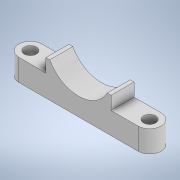
# Autodesk Inventor part: Стойка для заднего подшипника
Saved by Autodesk Inventor 2020 (Build 240168000, 168)
## iProperties
Created: 2021-04-13
Part Number: Стойка для заднего подшипника
Material: Типовые
Document SubType Name: Modeling
Designer: Антон
Density: 1 g/cm^3
Appearance: По умолчанию
Mass: 0.686339 g
Surface Area: 8.15331 cm^2
Volume: 0.686339 cm^3
Author: Антон
Autodesk Inventor part; units mm, degrees
ref_plane "YZ Plane" through (0, 0, 0) normal (1, 0, 0) x (0, 1, 0)
ref_plane "XZ Plane" through (0, 0, 0) normal (0, 1, 0) x (-1, 0, 0)
ref_plane "XY Plane" through (0, 0, 0) normal (0, 0, 1) x (1, 0, 0)
sketch "Эскиз6" plane through (0, 0, 0) normal (0, 0, 1) x (1, 0, 0)
  line L0 (0, 0) -> (10.05, 0)
  line L1 (10.05, 0) -> (10.05, 2)
  line L2 (10.05, 2) -> (0, 2)
  line L3 (0, 2) -> (0, 0)
  line L4 (10.05, 0) -> (27.05, 0)
  line L5 (27.05, 0) -> (27.05, 9.55)
  line L6 (27.05, 9.55) -> (10.05, 9.55)
  line L7 (10.05, 9.55) -> (10.05, 0)
  line L8 (27.05, 0) -> (37.1, 0)
  line L9 (37.1, 0) -> (37.1, 2)
  line L10 (37.1, 2) -> (27.05, 2)
  line L11 (27.05, 2) -> (27.05, 0)
  line L12 (10.05, 5.4448) -> (11.05, 5.4448)
  line L13 (27.05, 5.4448) -> (26.05, 5.4448)
  circle A0 centre (18.55, 9.55) radius 8.55
  line L14 (0, 0) -> (37.1, 0)
  line L15 (37.1, 0) -> (37.1, -3.7)
  line L16 (37.1, -3.7) -> (0, -3.7)
  line L17 (0, -3.7) -> (0, 0)
  point P0 (10.05, 2)
  dimension "d20" = 10.05
  dimension "d21" = 2
  dimension "d22" = 17
  dimension "d23" = 9.55
  dimension "d29" = 1
  dimension "d30" = 1
  dimension "d31" = 17.1
  dimension "d42" = 3.7
  constraints: 36 end point, 8 parallel, 5 horizontal, 5 perpendicular, 2 equal length, 2 point on circle, 2 point on line, 1 centre point, 1 midpoint
  measures "d20" distance of L2.end L1.end
  measures "d21" distance of L1.end L0.end
  measures "d22" distance of L6.end L5.end
  measures "d23" distance of L5.end L4.end
  measures "d29" distance of L12.start L12.end
  measures "d30" distance of L13.start L13.end
  measures "d31" diameter of A0
  measures "d42" distance of L14.end L15.end
extrude "Выдавливание4" add sketch "Эскиз6" along normal blind 6 contours L3 L2 L1 L0 | L0 L4 L8 L15 L16 L17 | L1 L7 L12 A0 L13 L5 L4 | L5 L10 L9 L8
sketch "Эскиз7" plane through (0, 2, 0) normal (0, 1, 0) x (1, 0, 0)
  line L0 (0, 0) -> (0, -6) projected
  line L1 (0, -3) -> (3, -3)
  line L2 (37.1, 0) -> (37.1, -6) projected
  line L3 (37.1, -3) -> (34.1, -3)
  dimension "d32" = 3
  constraints: 4 end point, 2 horizontal, 2 midpoint, 1 collinear
  measures "d32" distance of L1.start L1.end
hole "Отверстие2" at (3, 2, 3) at (34.1, 2, 3) direction (0, -1, 0) diameter 3.2 end through all
fillet "Сопряжение1" radius 3 4 edges at (0, -0.85, 6) (0, -0.85, 0) (37.1, -0.85, 6) (37.1, -0.85, 0)
equation "\"d29\" = d30"
